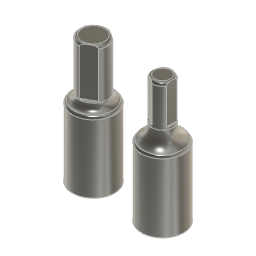
_Sanding adapters.f5689395-9ade-4c4c-a308-131110bf233c (Autodesk Fusion 360 design; units mm, degrees)
Autodesk Fusion 360 part; units mm, degrees
sketch "Sketch1" plane through (0, 0, 0) normal (0, 1, 0) x (1, 0, 0)
  line L0 (0, 0) -> (6.35, 0)
  line L1 (6.35, 0) -> (6.35, -25.4)
  line L2 (6.35, -25.4) -> (0, -25.4)
  line L3 (0, -25.4) -> (0, 0)
  line L4 (6.35, 0) -> (9.525, 0)
  line L5 (9.525, 0) -> (9.525, -25.4113)
  line L6 (9.525, -25.4113) -> (6.35, -25.4113)
  line L7 (6.35, -25.4113) -> (6.35, 0)
  line L8 (9.525, -25.4113) -> (0.0275, -25.4113)
  line L9 (0.0275, -25.4113) -> (0.0275, -31.7613)
  line L10 (0.0275, -31.7613) -> (9.525, -31.7613)
  line L11 (9.525, -31.7613) -> (9.525, -25.4113)
  line L12 (0.0275, -31.7613) -> (4.79, -31.7613)
  line L13 (4.79, -31.7613) -> (4.79, -57.15)
  line L14 (4.79, -57.15) -> (0.0275, -57.15)
  line L15 (0.0275, -57.15) -> (0.0275, -31.7613)
  arc A0 (9.525, -31.7613) -> (4.79, -38.8053) centre (12.397, -38.8053) ccw
  dimension "d1" = 6.35
  dimension "d2" = 25.4
  dimension "d3" = 3.175
  dimension "d4" = 6.35
  dimension "d5" = 4.7625
  constraint horizontal L0
  constraint vertical L1
  constraint horizontal L2
  constraint vertical L3
  constraint coincident L0.start L3.end
  constraint horizontal L4
  constraint vertical L5
  constraint horizontal L6
  constraint vertical L7
  constraint horizontal L8
  constraint vertical L9
  constraint horizontal L10
  constraint vertical L11
  constraint horizontal L12
  constraint vertical L13
  constraint horizontal L14
  constraint vertical L15
  constraint tangent L13 A0
  constraint coincident L13 A0.end
  measures "d1" distance of L0.start L0.end
  measures "d2" distance of L0.start L2.end
  measures "d3" distance of L0.end L4.end
  measures "d4" distance of L5.end L10.end
  measures "d5" distance of L9.end L12.end
revolve "Revolve1" add sketch "Sketch1" angle 360 about axis through (0.0275, 0, 57.15) along (0, 0, -1) contours L1 L4 L5 L6 L7 L8 | L6 L8 L9 L10 L11 L12 | L10 L13 A0 | L10 L12 L13 L14 L15 makes body 1
fillet "Fillet1" radius 0.254 2 edges at (-8.8273, -3.4344, 0) (-5.8671, -2.2863, 0) on bodies 1
fillet "Fillet2" radius 1.27 1 edges at (-8.8273, -3.4344, 31.7613) 1 faces at (0.6075, 0.1002, 57.15) on bodies 1
sketch "Sketch2" plane through (0, 0, 0) normal (0, 1, 0) x (1, 0, 0)
  line L0 (0.0275, -57.15) -> (0.0275, -31.7613)
  line L1 (0.0275, -25.4113) -> (0.0275, -31.7613)
  line L2 (6.35, -25.4) -> (0, -25.4)
  line L3 (6.35, -25.4113) -> (6.35, 0)
  line L4 (6.35, 0) -> (9.525, 0)
  line L5 (9.525, 0) -> (9.525, -25.4113)
  line L6 (9.525, -31.7613) -> (9.525, -25.4113)
  line L7 (0.0275, -57.15) -> (6.3775, -57.15)
  line L8 (6.3775, -57.15) -> (6.3775, -35.007)
  arc A0 (9.525, -31.7613) -> (6.3775, -35.007) centre (9.6247, -35.007) ccw
  line L9 (0.0275, -57.15) -> (6.3775, -57.15)
  line L10 (9.525, -31.7613) -> (0.0275, -31.7613)
  line L11 (9.525, -31.7613) -> (9.525, 0)
  dimension "d11" = 6.35
  constraint coincident L0.start L7.start
  constraint perpendicular L0 L7
  constraint perpendicular L7 L8
  constraint tangent L8 A0
  constraint coincident L6.start A0.start
  constraint coincident L0.end L1.end
  constraint coincident L4.end L5.start
  measures "d11" distance of L0.start L7.end
revolve "Revolve1'" add sketch "Sketch1" sketch "Sketch2" angle 360 about axis through (0.0275, 0, 57.15) along (0, 0, -1) separate body contours L1 L4 L5 L6 L7 L8 | L6 L8 L9 L10 L11 L12 of sketch 2 makes body 2 in component "Component"
fillet "Fillet1'" radius 1.27 1 edges at (-5.8928, -2.2963, 57.15) 2 faces at (9.3272, 0.9306, 31.7695) (6.3696, 0.3165, 49.769) on bodies 2 in component "Component"
fillet "Fillet2'" radius 0.254 2 edges at (-8.8273, -3.4344, 0) (-5.8671, -2.2863, 0) on bodies 2 in component "Component"
sketch "Sketch3" plane through (0, 0, 61.5242) normal (0, 0, 1) x (-1, 0, 0)
  circle A0 centre (33.2164, 0) radius 5.08
  circle A1 centre (33.2164, 0) radius 6.35
  circle A2 centre (33.2164, 0) radius 5.08
  circle A3 centre (-0.0275, 0) radius 4.7625
  circle A4 centre (-0.0275, 0) radius 3.4925
  line L0 (33.2164, -6.35) -> (38.7156, -3.175)
  line L1 (38.7156, -3.175) -> (38.7156, 3.175)
  line L2 (38.7156, 3.175) -> (33.2164, 6.35)
  line L3 (33.2164, 6.35) -> (27.7171, 3.175)
  line L4 (27.7171, 3.175) -> (27.7171, -3.175)
  line L5 (27.7171, -3.175) -> (33.2164, -6.35)
  line L6 (-0.0275, -4.7625) -> (4.0969, -2.3813)
  line L7 (4.0969, -2.3813) -> (4.0969, 2.3812)
  line L8 (4.0969, 2.3812) -> (-0.0275, 4.7625)
  line L9 (-0.0275, 4.7625) -> (-4.152, 2.3812)
  line L10 (-4.152, 2.3812) -> (-4.152, -2.3813)
  line L11 (-4.152, -2.3813) -> (-0.0275, -4.7625)
  point P0 (33.2164, 0)
  point P1 (-0.0275, 0)
  constraint coincident A1 L0.start
  constraint coincident P0 A0.centre
  constraint coincident A3 L6.start
  constraint coincident P1 A3.centre
extrude "Extrude1" cut sketch "Sketch3" against normal blind 21.59 contours A1 L1 | A1 L3 | A1 L5 | A3 L8 | A3 L6 | A3 L10 bodies 1
extrude "Extrude1'" cut sketch "Sketch3" against normal blind 21.59 contours A1 L1 | A1 L3 | A1 L5 | A3 L8 | A3 L6 | A3 L10 sketch seen with x (1, 0, 0) y (0, 1, 0) z (0, 0, 1) at (33.2439, 0, -4.3742) bodies 2 in component "Component"
component "Component" placed x (1, 0, 0) y (0, 1, 0) z (0, 0, 1) at (-33.2439, 0, 4.3742)
equation "d5 = ( 0.375 / 2 ) * 1 in"
